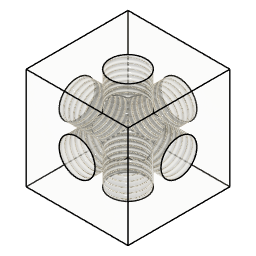
四方透明六面水晶螺母M4 (Autodesk Fusion 360 design; units mm, degrees)
Autodesk Fusion 360 part; units mm, degrees
sketch "草图1" plane through (0, 0, 0) normal (0, 0, 1) x (1, 0, 0)
  line L0 (0, 0) -> (10, 0)
  line L1 (10, 0) -> (10, 10)
  line L2 (10, 10) -> (0, 10)
  line L3 (0, 10) -> (0, 0)
  constraint horizontal L0
  constraint vertical L1
  constraint horizontal L2
  constraint vertical L3
  constraint coincident L0.start L3.end
extrude "拉伸1" add sketch "草图1" along normal blind 10
hole "孔1" at (5, 5, 10) direction (0, 0, -1) diameter 3.529 depth 10 tip angle 180
thread "螺纹1" "ISO Metric profile 4.0 M4x0.5 M4x0.5 6H" thread offset 0 thread depth 7.4
hole "孔2" at (0, 5, 5) direction (1, 0, 0) diameter 3.529 depth 5 tip angle 180
thread "螺纹2" "ISO Metric profile 4.0 M4x0.5 M4x0.5 6H" thread offset 0 thread depth 7.4
hole "孔3" at (10, 5, 5) direction (-1, 0, 0) diameter 3.529 depth 5 tip angle 180
thread "螺纹3" "ISO Metric profile 4.0 M4x0.5 M4x0.5 6H" thread offset 0 thread depth 7.4
hole "孔4" at (5, 10, 5) direction (0, -1, 0) diameter 3.529 depth 5 tip angle 180
thread "螺纹4" "ISO Metric profile 4.0 M4x0.5 M4x0.5 6H" thread offset 0 thread depth 7.4
hole "孔5" at (5, 0, 5) direction (0, 1, 0) diameter 3.529 depth 5 tip angle 180
thread "螺纹5" "ISO Metric profile 4.0 M4x0.5 M4x0.5 6H" thread offset 0 thread depth 7.4
